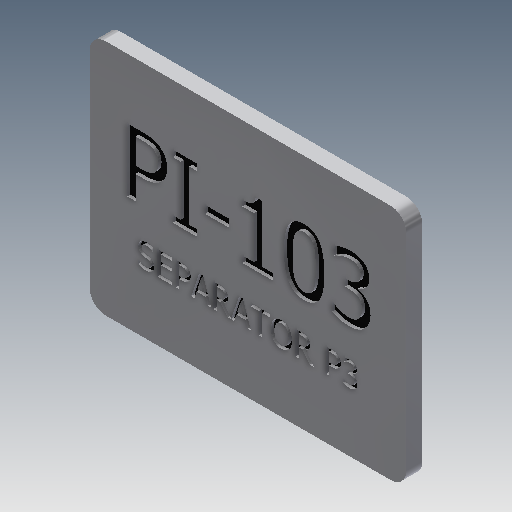
# Autodesk Inventor part: PI-103_Instrument Name Plate
Saved by Autodesk Inventor 2019.1 (Build 231200000, 200)
## iProperties
Created: 2009-08-11
Part Number: PI-103_Instrument Name Plate
Material: Polyaryletherketone Resin
Document SubType Name: Modeling
Designer: Demir Ali
Mass: 48.4644 g
Surface Area: 174.794 cm^2
Volume: 36.7154 cm^3
Density: 1.32 g/cm^3
Description: Name Plate
Stock Number: NA
Appearance: Smooth - White
Title: Purchased Part
Author: Demir Ali
Revision Number: A
Autodesk Inventor part; units mm, degrees
ref_plane "YZ Plane" through (0, 0, 0) normal (1, 0, 0) x (0, 1, 0)
ref_plane "XZ Plane" through (0, 0, 0) normal (0, 1, 0) x (-1, 0, 0)
ref_plane "XY Plane" through (0, 0, 0) normal (0, 0, 1) x (1, 0, 0)
sketch "Sketch1" plane through (0, 0, 0) normal (0, 0, 1) x (1, 0, 0)
  line L0 (-50, -37.5) -> (50, -37.5)
  line L1 (50, -37.5) -> (50, 37.5)
  line L2 (50, 37.5) -> (-50, 37.5)
  line L3 (-50, 37.5) -> (-50, -37.5)
  point P0 (0, 0)
  point P1 (50, 0)
  point P2 (0, 37.5)
  dimension "d0" = 100
  dimension "d1" = 75
  constraints: 8 end point, 2 midpoint, 2 parallel, 1 horizontal, 1 horizontal alignment, 1 perpendicular, 1 vertical alignment
  measures "d0" distance of L1.end L2.end
  measures "d1" distance of L0.end L1.end
extrude "Extrusion1" add sketch "Sketch1" along normal blind 5
sketch "Sketch2" plane through (0, 0, 5) normal (0, 0, 1) x (1, 0, 0)
  line L0 (-39.7109, 33.8079) -> (39.7109, 33.8079) construction
  line L1 (39.7109, 33.8079) -> (39.7109, -33.8079) construction
  line L2 (39.7109, -33.8079) -> (-39.7109, -33.8079) construction
  line L3 (-39.7109, -33.8079) -> (-39.7109, 33.8079) construction
  line L4 (-50, -37.5) -> (-50, 37.5) projected
  line L5 (50, -37.5) -> (-50, -37.5) projected
  line L6 (50, 37.5) -> (50, -37.5) projected
  line L7 (-50, 37.5) -> (50, 37.5) projected
  spline S0 degree 2 poles (-25.5511, 12.4253) (-25.5511, 11.1287) (-26.4749, 8.7948) (-27.3015, 7.9844) knots 0 0 0 1 2 2 2
  spline S1 degree 2 poles (-27.3015, 7.9844) (-28.3387, 6.9633) (-31.1426, 5.9099) (-33.282, 5.9099) knots 0 0 0 1 2 2 2
  line L8 (-33.282, 5.9099) -> (-35.5348, 5.9099)
  line L9 (-35.5348, 5.9099) -> (-35.5348, -1.5456)
  line L10 (-35.5348, -1.5456) -> (-38.1929, -1.5456)
  line L11 (-38.1929, -1.5456) -> (-38.1929, 18.4544)
  line L12 (-38.1929, 18.4544) -> (-33.1686, 18.4544)
  spline S2 degree 2 poles (-33.1686, 18.4544) (-31.3857, 18.4544) (-28.8898, 17.871) (-27.9336, 17.2065) knots 0 0 0 1 2 2 2
  spline S3 degree 2 poles (-27.9336, 17.2065) (-26.8152, 16.4447) (-25.5511, 14.0946) (-25.5511, 12.4253) knots 0 0 0 1 2 2 2
  spline S4 degree 2 poles (-28.3225, 12.3442) (-28.3225, 13.3815) (-29.0357, 14.905) (-29.765, 15.3912) knots 0 0 0 1 2 2 2
  spline S5 degree 2 poles (-29.765, 15.3912) (-30.3971, 15.8126) (-32.0827, 16.153) (-33.3306, 16.153) knots 0 0 0 1 2 2 2
  line L13 (-33.3306, 16.153) -> (-35.5348, 16.153)
  line L14 (-35.5348, 16.153) -> (-35.5348, 8.1789)
  line L15 (-35.5348, 8.1789) -> (-33.7196, 8.1789)
  spline S6 degree 2 poles (-33.7196, 8.1789) (-32.0989, 8.1789) (-30.1053, 8.6975) (-29.4571, 9.3783) knots 0 0 0 1 2 2 2
  spline S7 degree 2 poles (-29.4571, 9.3783) (-28.8574, 9.9779) (-28.3225, 11.388) (-28.3225, 12.3442) knots 0 0 0 1 2 2 2
  line L16 (-16.0535, -1.5456) -> (-23.8006, -1.5456)
  line L17 (-23.8006, -1.5456) -> (-23.8006, 0.4966)
  line L18 (-23.8006, 0.4966) -> (-21.2561, 0.4966)
  line L19 (-21.2561, 0.4966) -> (-21.2561, 16.4123)
  line L20 (-21.2561, 16.4123) -> (-23.8006, 16.4123)
  line L21 (-23.8006, 16.4123) -> (-23.8006, 18.4544)
  line L22 (-23.8006, 18.4544) -> (-16.0535, 18.4544)
  line L23 (-16.0535, 18.4544) -> (-16.0535, 16.4123)
  line L24 (-16.0535, 16.4123) -> (-18.5981, 16.4123)
  line L25 (-18.5981, 16.4123) -> (-18.5981, 0.4966)
  line L26 (-18.5981, 0.4966) -> (-16.0535, 0.4966)
  line L27 (-16.0535, 0.4966) -> (-16.0535, -1.5456)
  line L28 (-6.0049, 5.9909) -> (-13.5737, 5.9909)
  line L29 (-13.5737, 5.9909) -> (-13.5737, 8.422)
  line L30 (-13.5737, 8.422) -> (-6.0049, 8.422)
  line L31 (-6.0049, 8.422) -> (-6.0049, 5.9909)
  line L32 (7.9822, -1.5456) -> (-1.7747, -1.5456)
  line L33 (-1.7747, -1.5456) -> (-1.7747, 0.4966)
  line L34 (-1.7747, 0.4966) -> (1.8558, 0.4966)
  line L35 (1.8558, 0.4966) -> (1.8558, 13.9001)
  line L36 (1.8558, 13.9001) -> (-1.7747, 13.9001)
  line L37 (-1.7747, 13.9001) -> (-1.7747, 15.7316)
  spline S8 degree 2 poles (-1.7747, 15.7316) (0.2836, 15.7316) (2.2285, 16.8985) (2.3582, 18.5193) knots 0 0 0 1 2 2 2
  line L38 (2.3582, 18.5193) -> (4.4327, 18.5193)
  line L39 (4.4327, 18.5193) -> (4.4327, 0.4966)
  line L40 (4.4327, 0.4966) -> (7.9822, 0.4966)
  line L41 (7.9822, 0.4966) -> (7.9822, -1.5456)
  spline S9 degree 2 poles (24.1086, 8.4544) (24.1086, 3.0736) (20.9806, -1.967) (17.7229, -1.967) knots 0 0 0 1 2 2 2
  spline S10 degree 2 poles (17.7229, -1.967) (14.4165, -1.967) (11.3209, 3.1708) (11.3209, 8.4382) knots 0 0 0 1 2 2 2
  spline S11 degree 2 poles (11.3209, 8.4382) (11.3209, 13.8515) (14.4489, 18.8596) (17.7229, 18.8596) knots 0 0 0 1 2 2 2
  spline S12 degree 2 poles (17.7229, 18.8596) (21.013, 18.8596) (24.1086, 13.6732) (24.1086, 8.4544) knots 0 0 0 1 2 2 2
  spline S13 degree 2 poles (20.6726, 2.3604) (21.0616, 3.3491) (21.3857, 6.3961) (21.3857, 8.4544) knots 0 0 0 1 2 2 2
  spline S14 degree 2 poles (21.3857, 8.4544) (21.3857, 10.5128) (21.0616, 13.5436) (20.6564, 14.5646) knots 0 0 0 1 2 2 2
  spline S15 degree 2 poles (20.6564, 14.5646) (20.2512, 15.5857) (18.8412, 16.6392) (17.7229, 16.6392) knots 0 0 0 1 2 2 2
  spline S16 degree 2 poles (17.7229, 16.6392) (16.6045, 16.6392) (15.1621, 15.5857) (14.7407, 14.5322) knots 0 0 0 1 2 2 2
  spline S17 degree 2 poles (14.7407, 14.5322) (14.3355, 13.5112) (14.0438, 10.3993) (14.0438, 8.4382) knots 0 0 0 1 2 2 2
  spline S18 degree 2 poles (14.0438, 8.4382) (14.0438, 6.3313) (14.3031, 3.5112) (14.7245, 2.4091) knots 0 0 0 1 2 2 2
  spline S19 degree 2 poles (14.7245, 2.4091) (15.1135, 1.3718) (16.5559, 0.2535) (17.7229, 0.2535) knots 0 0 0 1 2 2 2
  spline S20 degree 2 poles (17.7229, 0.2535) (18.825, 0.2535) (20.2674, 1.3069) (20.6726, 2.3604) knots 0 0 0 1 2 2 2
  spline S21 degree 2 poles (32.0664, 16.5582) (31.3371, 16.5582) (29.8947, 16.2016) (29.1977, 15.9261) knots 0 0 0 1 2 2 2
  spline S22 degree 2 poles (29.1977, 15.9261) (28.5494, 15.6505) (27.5932, 15.0671) (27.2204, 14.8078) knots 0 0 0 1 2 2 2
  line L42 (27.2204, 14.8078) -> (27.0583, 14.8078)
  line L43 (27.0583, 14.8078) -> (27.0583, 17.6441)
  spline S23 degree 2 poles (27.0583, 17.6441) (27.9335, 18.1141) (30.9319, 18.8758) (32.2771, 18.8758) knots 0 0 0 1 2 2 2
  spline S24 degree 2 poles (32.2771, 18.8758) (33.6386, 18.8758) (35.6645, 18.3248) (36.4911, 17.7413) knots 0 0 0 1 2 2 2
  spline S25 degree 2 poles (36.4911, 17.7413) (37.3663, 17.1092) (38.2739, 15.2778) (38.2739, 14.046) knots 0 0 0 1 2 2 2
  spline S26 degree 2 poles (38.2739, 14.046) (38.2739, 12.3928) (36.1021, 9.8969) (34.5786, 9.5727) knots 0 0 0 1 2 2 2
  line L44 (34.5786, 9.5727) -> (34.5786, 9.3783)
  spline S27 degree 2 poles (34.5786, 9.3783) (35.2107, 9.2486) (36.6532, 8.6651) (37.269, 8.0817) knots 0 0 0 1 2 2 2
  spline S28 degree 2 poles (37.269, 8.0817) (37.8849, 7.5144) (38.6629, 5.6992) (38.6629, 4.3864) knots 0 0 0 1 2 2 2
  spline S29 degree 2 poles (38.6629, 4.3864) (38.6629, 3.0411) (37.7391, 0.7559) (36.8963, -0.1193) knots 0 0 0 1 2 2 2
  spline S30 degree 2 poles (36.8963, -0.1193) (36.0211, -1.0269) (33.5413, -1.967) (31.9692, -1.967) knots 0 0 0 1 2 2 2
  spline S31 degree 2 poles (31.9692, -1.967) (30.4619, -1.967) (27.5122, -1.2376) (26.5073, -0.7352) knots 0 0 0 1 2 2 2
  line L45 (26.5073, -0.7352) -> (26.5073, 2.1011)
  line L46 (26.5073, 2.1011) -> (26.7018, 2.1011)
  spline S32 degree 2 poles (26.7018, 2.1011) (27.5446, 1.4852) (30.3971, 0.3507) (31.8071, 0.3507) knots 0 0 0 1 2 2 2
  spline S33 degree 2 poles (31.8071, 0.3507) (32.6337, 0.3507) (34.2869, 0.8693) (34.8379, 1.469) knots 0 0 0 1 2 2 2
  spline S34 degree 2 poles (34.8379, 1.469) (35.3728, 2.0687) (35.94, 3.495) (35.94, 4.5809) knots 0 0 0 1 2 2 2
  spline S35 degree 2 poles (35.94, 4.5809) (35.94, 5.6668) (35.3079, 7.0768) (34.7407, 7.482) knots 0 0 0 1 2 2 2
  spline S36 degree 2 poles (34.7407, 7.482) (34.1734, 7.8872) (32.6337, 8.1951) (31.7261, 8.1951) knots 0 0 0 1 2 2 2
  line L47 (31.7261, 8.1951) -> (30.5916, 8.1951)
  line L48 (30.5916, 8.1951) -> (30.5916, 10.4155)
  line L49 (30.5916, 10.4155) -> (31.483, 10.4155)
  spline S37 degree 2 poles (31.483, 10.4155) (33.282, 10.4155) (35.5511, 12.1335) (35.5511, 13.7705) knots 0 0 0 1 2 2 2
  spline S38 degree 2 poles (35.5511, 13.7705) (35.5511, 14.5322) (34.9676, 15.6181) (34.4976, 15.9423) knots 0 0 0 1 2 2 2
  spline S39 degree 2 poles (34.4976, 15.9423) (33.9951, 16.2826) (32.7634, 16.5582) (32.0664, 16.5582) knots 0 0 0 1 2 2 2
  spline S40 degree 2 poles (-32.2761, -18.8515) (-33.0906, -18.8515) (-34.2332, -18.5112) (-34.7376, -18.268) knots 0 0 0 1 2 2 2
  line L50 (-34.7376, -18.268) -> (-34.7376, -17.016)
  line L51 (-34.7376, -17.016) -> (-34.6647, -17.016)
  spline S41 degree 2 poles (-34.6647, -17.016) (-34.1724, -17.4779) (-32.9265, -17.9885) (-32.3491, -17.9885) knots 0 0 0 1 2 2 2
  spline S42 degree 2 poles (-32.3491, -17.9885) (-31.5225, -17.9885) (-30.6777, -17.3017) (-30.6777, -16.7364) knots 0 0 0 1 2 2 2
  spline S43 degree 2 poles (-30.6777, -16.7364) (-30.6777, -16.2867) (-31.1214, -15.7275) (-31.6015, -15.5877) knots 0 0 0 1 2 2 2
  spline S44 degree 2 poles (-31.6015, -15.5877) (-31.9479, -15.4905) (-32.5253, -15.3568) (-32.9568, -15.2474) knots 0 0 0 1 2 2 2
  spline S45 degree 2 poles (-32.9568, -15.2474) (-33.3458, -15.1441) (-33.9597, -14.8341) (-34.1967, -14.5849) knots 0 0 0 1 2 2 2
  spline S46 degree 2 poles (-34.1967, -14.5849) (-34.4277, -14.3357) (-34.6829, -13.6672) (-34.6829, -13.2296) knots 0 0 0 1 2 2 2
  spline S47 degree 2 poles (-34.6829, -13.2296) (-34.6829, -12.3179) (-33.2607, -11.0841) (-32.1607, -11.0841) knots 0 0 0 1 2 2 2
  spline S48 degree 2 poles (-32.1607, -11.0841) (-31.5286, -11.0841) (-30.4103, -11.3333) (-29.9301, -11.5703) knots 0 0 0 1 2 2 2
  line L52 (-29.9301, -11.5703) -> (-29.9301, -12.7616)
  line L53 (-29.9301, -12.7616) -> (-30.003, -12.7616)
  spline S49 degree 2 poles (-30.003, -12.7616) (-30.3616, -12.4334) (-31.4799, -11.9471) (-32.0938, -11.9471) knots 0 0 0 1 2 2 2
  spline S50 degree 2 poles (-32.0938, -11.9471) (-32.7867, -11.9471) (-33.6436, -12.5975) (-33.6436, -13.1262) knots 0 0 0 1 2 2 2
  spline S51 degree 2 poles (-33.6436, -13.1262) (-33.6436, -13.6003) (-33.1392, -14.1655) (-32.6651, -14.2932) knots 0 0 0 1 2 2 2
  spline S52 degree 2 poles (-32.6651, -14.2932) (-32.3491, -14.3783) (-31.4313, -14.5971) (-31.1274, -14.6882) knots 0 0 0 1 2 2 2
  spline S53 degree 2 poles (-31.1274, -14.6882) (-30.3556, -14.9253) (-29.6384, -15.8795) (-29.6384, -16.5784) knots 0 0 0 1 2 2 2
  spline S54 degree 2 poles (-29.6384, -16.5784) (-29.6384, -17.0221) (-29.997, -17.873) (-30.3191, -18.1708) knots 0 0 0 1 2 2 2
  spline S55 degree 2 poles (-30.3191, -18.1708) (-30.6777, -18.499) (-31.5893, -18.8515) (-32.2761, -18.8515) knots 0 0 0 1 2 2 2
  line L54 (-28.6234, -18.7178) -> (-28.6234, -11.2178)
  line L55 (-28.6234, -11.2178) -> (-23.9313, -11.2178)
  line L56 (-23.9313, -11.2178) -> (-23.9313, -12.1052)
  line L57 (-23.9313, -12.1052) -> (-27.6266, -12.1052)
  line L58 (-27.6266, -12.1052) -> (-27.6266, -14.1595)
  line L59 (-27.6266, -14.1595) -> (-24.1805, -14.1595)
  line L60 (-24.1805, -14.1595) -> (-24.1805, -15.0468)
  line L61 (-24.1805, -15.0468) -> (-27.6266, -15.0468)
  line L62 (-27.6266, -15.0468) -> (-27.6266, -17.8304)
  line L63 (-27.6266, -17.8304) -> (-23.9313, -17.8304)
  line L64 (-23.9313, -17.8304) -> (-23.9313, -18.7178)
  line L65 (-23.9313, -18.7178) -> (-28.6234, -18.7178)
  spline S56 degree 2 poles (-18.0966, -13.4787) (-18.0966, -13.965) (-18.4431, -14.8402) (-18.753, -15.1441) knots 0 0 0 1 2 2 2
  spline S57 degree 2 poles (-18.753, -15.1441) (-19.142, -15.527) (-20.1935, -15.922) (-20.9957, -15.922) knots 0 0 0 1 2 2 2
  line L66 (-20.9957, -15.922) -> (-21.8406, -15.922)
  line L67 (-21.8406, -15.922) -> (-21.8406, -18.7178)
  line L68 (-21.8406, -18.7178) -> (-22.8373, -18.7178)
  line L69 (-22.8373, -18.7178) -> (-22.8373, -11.2178)
  line L70 (-22.8373, -11.2178) -> (-20.9532, -11.2178)
  spline S58 degree 2 poles (-20.9532, -11.2178) (-20.2846, -11.2178) (-19.3487, -11.4366) (-18.9901, -11.6858) knots 0 0 0 1 2 2 2
  spline S59 degree 2 poles (-18.9901, -11.6858) (-18.5707, -11.9714) (-18.0966, -12.8527) (-18.0966, -13.4787) knots 0 0 0 1 2 2 2
  spline S60 degree 2 poles (-19.1359, -13.5091) (-19.1359, -13.1202) (-19.4034, -12.5488) (-19.6769, -12.3665) knots 0 0 0 1 2 2 2
  spline S61 degree 2 poles (-19.6769, -12.3665) (-19.9139, -12.2085) (-20.546, -12.0808) (-21.014, -12.0808) knots 0 0 0 1 2 2 2
  line L71 (-21.014, -12.0808) -> (-21.8406, -12.0808)
  line L72 (-21.8406, -12.0808) -> (-21.8406, -15.0711)
  line L73 (-21.8406, -15.0711) -> (-21.1598, -15.0711)
  spline S62 degree 2 poles (-21.1598, -15.0711) (-20.5521, -15.0711) (-19.8045, -14.8766) (-19.5614, -14.6214) knots 0 0 0 1 2 2 2
  spline S63 degree 2 poles (-19.5614, -14.6214) (-19.3365, -14.3965) (-19.1359, -13.8677) (-19.1359, -13.5091) knots 0 0 0 1 2 2 2
  line L74 (-17.9568, -18.7178) -> (-15.4285, -11.2178)
  line L75 (-15.4285, -11.2178) -> (-14.2008, -11.2178)
  line L76 (-14.2008, -11.2178) -> (-11.6724, -18.7178)
  line L77 (-11.6724, -18.7178) -> (-12.7239, -18.7178)
  line L78 (-12.7239, -18.7178) -> (-13.4046, -16.621)
  line L79 (-13.4046, -16.621) -> (-16.2672, -16.621)
  line L80 (-16.2672, -16.621) -> (-16.9479, -18.7178)
  line L81 (-16.9479, -18.7178) -> (-17.9568, -18.7178)
  line L82 (-13.6781, -15.7701) -> (-14.8389, -12.2389)
  line L83 (-14.8389, -12.2389) -> (-15.9937, -15.7701)
  line L84 (-15.9937, -15.7701) -> (-13.6781, -15.7701)
  line L85 (-5.157, -18.7178) -> (-6.4516, -18.7178)
  line L86 (-6.4516, -18.7178) -> (-8.8219, -15.7336)
  line L87 (-8.8219, -15.7336) -> (-9.9645, -15.7336)
  line L88 (-9.9645, -15.7336) -> (-9.9645, -18.7178)
  line L89 (-9.9645, -18.7178) -> (-10.9613, -18.7178)
  line L90 (-10.9613, -18.7178) -> (-10.9613, -11.2178)
  line L91 (-10.9613, -11.2178) -> (-9.0286, -11.2178)
  spline S64 degree 2 poles (-9.0286, -11.2178) (-8.3843, -11.2178) (-7.5152, -11.3576) (-7.1201, -11.6129) knots 0 0 0 1 2 2 2
  spline S65 degree 2 poles (-7.1201, -11.6129) (-6.7251, -11.8681) (-6.2692, -12.6643) (-6.2692, -13.2539) knots 0 0 0 1 2 2 2
  spline S66 degree 2 poles (-6.2692, -13.2539) (-6.2692, -14.0744) (-7.108, -15.1866) (-7.8252, -15.454) knots 0 0 0 1 2 2 2
  line L92 (-7.8252, -15.454) -> (-5.157, -18.7178)
  spline S67 degree 2 poles (-7.3086, -13.3329) (-7.3086, -13.0047) (-7.5395, -12.5002) (-7.7826, -12.3361) knots 0 0 0 1 2 2 2
  spline S68 degree 2 poles (-7.7826, -12.3361) (-7.9953, -12.1963) (-8.5606, -12.0808) (-8.9739, -12.0808) knots 0 0 0 1 2 2 2
  line L93 (-8.9739, -12.0808) -> (-9.9645, -12.0808)
  line L94 (-9.9645, -12.0808) -> (-9.9645, -14.9009)
  line L95 (-9.9645, -14.9009) -> (-9.0893, -14.9009)
  spline S69 degree 2 poles (-9.0893, -14.9009) (-8.6578, -14.9009) (-7.971, -14.749) (-7.734, -14.512) knots 0 0 0 1 2 2 2
  spline S70 degree 2 poles (-7.734, -14.512) (-7.5152, -14.3053) (-7.3086, -13.7219) (-7.3086, -13.3329) knots 0 0 0 1 2 2 2
  line L96 (-5.3697, -18.7178) -> (-2.8414, -11.2178)
  line L97 (-2.8414, -11.2178) -> (-1.6137, -11.2178)
  line L98 (-1.6137, -11.2178) -> (0.9147, -18.7178)
  line L99 (0.9147, -18.7178) -> (-0.1368, -18.7178)
  line L100 (-0.1368, -18.7178) -> (-0.8175, -16.621)
  line L101 (-0.8175, -16.621) -> (-3.6801, -16.621)
  line L102 (-3.6801, -16.621) -> (-4.3608, -18.7178)
  line L103 (-4.3608, -18.7178) -> (-5.3697, -18.7178)
  line L104 (-1.091, -15.7701) -> (-2.2518, -12.2389)
  line L105 (-2.2518, -12.2389) -> (-3.4066, -15.7701)
  line L106 (-3.4066, -15.7701) -> (-1.091, -15.7701)
  line L107 (3.3762, -18.7178) -> (3.3762, -12.1052)
  line L108 (3.3762, -12.1052) -> (0.86, -12.1052)
  line L109 (0.86, -12.1052) -> (0.86, -11.2178)
  line L110 (0.86, -11.2178) -> (6.8892, -11.2178)
  line L111 (6.8892, -11.2178) -> (6.8892, -12.1052)
  line L112 (6.8892, -12.1052) -> (4.373, -12.1052)
  line L113 (4.373, -12.1052) -> (4.373, -18.7178)
  line L114 (4.373, -18.7178) -> (3.3762, -18.7178)
  spline S71 degree 2 poles (12.9548, -12.0748) (13.3803, -12.5732) (13.8543, -14.0318) (13.8543, -14.9678) knots 0 0 0 1 2 2 2
  spline S72 degree 2 poles (13.8543, -14.9678) (13.8543, -15.8795) (13.3924, -17.3564) (12.9548, -17.8548) knots 0 0 0 1 2 2 2
  spline S73 degree 2 poles (12.9548, -17.8548) (12.4929, -18.3774) (11.2713, -18.8758) (10.5359, -18.8758) knots 0 0 0 1 2 2 2
  spline S74 degree 2 poles (10.5359, -18.8758) (9.7761, -18.8758) (8.5606, -18.3592) (8.1169, -17.8548) knots 0 0 0 1 2 2 2
  spline S75 degree 2 poles (8.1169, -17.8548) (7.6854, -17.3564) (7.2235, -15.8916) (7.2235, -14.9678) knots 0 0 0 1 2 2 2
  spline S76 degree 2 poles (7.2235, -14.9678) (7.2235, -14.0257) (7.6914, -12.5914) (8.123, -12.0748) knots 0 0 0 1 2 2 2
  spline S77 degree 2 poles (8.123, -12.0748) (8.5606, -11.5764) (9.7822, -11.0598) (10.5359, -11.0598) knots 0 0 0 1 2 2 2
  spline S78 degree 2 poles (10.5359, -11.0598) (11.3017, -11.0598) (12.5294, -11.5946) (12.9548, -12.0748) knots 0 0 0 1 2 2 2
  spline S79 degree 2 poles (12.815, -14.9678) (12.815, -14.2263) (12.4929, -13.0776) (12.2012, -12.7008) knots 0 0 0 1 2 2 2
  spline S80 degree 2 poles (12.2012, -12.7008) (11.9034, -12.3118) (11.0646, -11.9228) (10.5419, -11.9228) knots 0 0 0 1 2 2 2
  spline S81 degree 2 poles (10.5419, -11.9228) (10.001, -11.9228) (9.1866, -12.2997) (8.8766, -12.7008) knots 0 0 0 1 2 2 2
  spline S82 degree 2 poles (8.8766, -12.7008) (8.5788, -13.0837) (8.2628, -14.2385) (8.2628, -14.9678) knots 0 0 0 1 2 2 2
  spline S83 degree 2 poles (8.2628, -14.9678) (8.2628, -16.4447) (9.5026, -18.0128) (10.5419, -18.0128) knots 0 0 0 1 2 2 2
  spline S84 degree 2 poles (10.5419, -18.0128) (11.5812, -18.0128) (12.815, -16.4447) (12.815, -14.9678) knots 0 0 0 1 2 2 2
  line L115 (20.7526, -18.7178) -> (19.4581, -18.7178)
  line L116 (19.4581, -18.7178) -> (17.0877, -15.7336)
  line L117 (17.0877, -15.7336) -> (15.9451, -15.7336)
  line L118 (15.9451, -15.7336) -> (15.9451, -18.7178)
  line L119 (15.9451, -18.7178) -> (14.9483, -18.7178)
  line L120 (14.9483, -18.7178) -> (14.9483, -11.2178)
  line L121 (14.9483, -11.2178) -> (16.8811, -11.2178)
  spline S85 degree 2 poles (16.8811, -11.2178) (17.5253, -11.2178) (18.3944, -11.3576) (18.7895, -11.6129) knots 0 0 0 1 2 2 2
  spline S86 degree 2 poles (18.7895, -11.6129) (19.1846, -11.8681) (19.6404, -12.6643) (19.6404, -13.2539) knots 0 0 0 1 2 2 2
  spline S87 degree 2 poles (19.6404, -13.2539) (19.6404, -14.0744) (18.8017, -15.1866) (18.0845, -15.454) knots 0 0 0 1 2 2 2
  line L122 (18.0845, -15.454) -> (20.7526, -18.7178)
  spline S88 degree 2 poles (18.6011, -13.3329) (18.6011, -13.0047) (18.3701, -12.5002) (18.127, -12.3361) knots 0 0 0 1 2 2 2
  spline S89 degree 2 poles (18.127, -12.3361) (17.9143, -12.1963) (17.3491, -12.0808) (16.9358, -12.0808) knots 0 0 0 1 2 2 2
  line L123 (16.9358, -12.0808) -> (15.9451, -12.0808)
  line L124 (15.9451, -12.0808) -> (15.9451, -14.9009)
  line L125 (15.9451, -14.9009) -> (16.8203, -14.9009)
  spline S90 degree 2 poles (16.8203, -14.9009) (17.2518, -14.9009) (17.9386, -14.749) (18.1756, -14.512) knots 0 0 0 1 2 2 2
  spline S91 degree 2 poles (18.1756, -14.512) (18.3944, -14.3053) (18.6011, -13.7219) (18.6011, -13.3329) knots 0 0 0 1 2 2 2
  spline S92 degree 2 poles (29.3102, -13.4787) (29.3102, -13.965) (28.9637, -14.8402) (28.6538, -15.1441) knots 0 0 0 1 2 2 2
  spline S93 degree 2 poles (28.6538, -15.1441) (28.2648, -15.527) (27.2133, -15.922) (26.4111, -15.922) knots 0 0 0 1 2 2 2
  line L126 (26.4111, -15.922) -> (25.5662, -15.922)
  line L127 (25.5662, -15.922) -> (25.5662, -18.7178)
  line L128 (25.5662, -18.7178) -> (24.5695, -18.7178)
  line L129 (24.5695, -18.7178) -> (24.5695, -11.2178)
  line L130 (24.5695, -11.2178) -> (26.4536, -11.2178)
  spline S94 degree 2 poles (26.4536, -11.2178) (27.1222, -11.2178) (28.0581, -11.4366) (28.4167, -11.6858) knots 0 0 0 1 2 2 2
  spline S95 degree 2 poles (28.4167, -11.6858) (28.8361, -11.9714) (29.3102, -12.8527) (29.3102, -13.4787) knots 0 0 0 1 2 2 2
  spline S96 degree 2 poles (28.2709, -13.5091) (28.2709, -13.1202) (28.0034, -12.5488) (27.7299, -12.3665) knots 0 0 0 1 2 2 2
  spline S97 degree 2 poles (27.7299, -12.3665) (27.4929, -12.2085) (26.8608, -12.0808) (26.3928, -12.0808) knots 0 0 0 1 2 2 2
  line L131 (26.3928, -12.0808) -> (25.5662, -12.0808)
  line L132 (25.5662, -12.0808) -> (25.5662, -15.0711)
  line L133 (25.5662, -15.0711) -> (26.247, -15.0711)
  spline S98 degree 2 poles (26.247, -15.0711) (26.8547, -15.0711) (27.6023, -14.8766) (27.8454, -14.6214) knots 0 0 0 1 2 2 2
  spline S99 degree 2 poles (27.8454, -14.6214) (28.0703, -14.3965) (28.2709, -13.8677) (28.2709, -13.5091) knots 0 0 0 1 2 2 2
  spline S100 degree 2 poles (32.0695, -11.9289) (31.796, -11.9289) (31.2551, -12.0626) (30.9937, -12.1659) knots 0 0 0 1 2 2 2
  spline S101 degree 2 poles (30.9937, -12.1659) (30.7506, -12.2693) (30.392, -12.4881) (30.2522, -12.5853) knots 0 0 0 1 2 2 2
  line L134 (30.2522, -12.5853) -> (30.1914, -12.5853)
  line L135 (30.1914, -12.5853) -> (30.1914, -11.5217)
  spline S102 degree 2 poles (30.1914, -11.5217) (30.5197, -11.3454) (31.644, -11.0598) (32.1485, -11.0598) knots 0 0 0 1 2 2 2
  spline S103 degree 2 poles (32.1485, -11.0598) (32.659, -11.0598) (33.4188, -11.2664) (33.7287, -11.4852) knots 0 0 0 1 2 2 2
  spline S104 degree 2 poles (33.7287, -11.4852) (34.0569, -11.7223) (34.3973, -12.4091) (34.3973, -12.871) knots 0 0 0 1 2 2 2
  spline S105 degree 2 poles (34.3973, -12.871) (34.3973, -13.4909) (33.5829, -14.4269) (33.0115, -14.5484) knots 0 0 0 1 2 2 2
  line L136 (33.0115, -14.5484) -> (33.0115, -14.6214)
  spline S106 degree 2 poles (33.0115, -14.6214) (33.2486, -14.67) (33.7895, -14.8888) (34.0205, -15.1076) knots 0 0 0 1 2 2 2
  spline S107 degree 2 poles (34.0205, -15.1076) (34.2514, -15.3203) (34.5432, -16.001) (34.5432, -16.4933) knots 0 0 0 1 2 2 2
  spline S108 degree 2 poles (34.5432, -16.4933) (34.5432, -16.9978) (34.1967, -17.8548) (33.8807, -18.183) knots 0 0 0 1 2 2 2
  spline S109 degree 2 poles (33.8807, -18.183) (33.5525, -18.5233) (32.6226, -18.8758) (32.033, -18.8758) knots 0 0 0 1 2 2 2
  spline S110 degree 2 poles (32.033, -18.8758) (31.4678, -18.8758) (30.3616, -18.6023) (29.9848, -18.4139) knots 0 0 0 1 2 2 2
  line L137 (29.9848, -18.4139) -> (29.9848, -17.3503)
  line L138 (29.9848, -17.3503) -> (30.0577, -17.3503)
  spline S111 degree 2 poles (30.0577, -17.3503) (30.3738, -17.5813) (31.4435, -18.0067) (31.9722, -18.0067) knots 0 0 0 1 2 2 2
  spline S112 degree 2 poles (31.9722, -18.0067) (32.2822, -18.0067) (32.9021, -17.8122) (33.1088, -17.5873) knots 0 0 0 1 2 2 2
  spline S113 degree 2 poles (33.1088, -17.5873) (33.3094, -17.3625) (33.5221, -16.8276) (33.5221, -16.4204) knots 0 0 0 1 2 2 2
  spline S114 degree 2 poles (33.5221, -16.4204) (33.5221, -16.0132) (33.285, -15.4844) (33.0723, -15.3325) knots 0 0 0 1 2 2 2
  spline S115 degree 2 poles (33.0723, -15.3325) (32.8596, -15.1805) (32.2822, -15.065) (31.9419, -15.065) knots 0 0 0 1 2 2 2
  line L139 (31.9419, -15.065) -> (31.5164, -15.065)
  line L140 (31.5164, -15.065) -> (31.5164, -14.2324)
  line L141 (31.5164, -14.2324) -> (31.8507, -14.2324)
  spline S116 degree 2 poles (31.8507, -14.2324) (32.5253, -14.2324) (33.3762, -13.5881) (33.3762, -12.9743) knots 0 0 0 1 2 2 2
  spline S117 degree 2 poles (33.3762, -12.9743) (33.3762, -12.6886) (33.1574, -12.2814) (32.9812, -12.1599) knots 0 0 0 1 2 2 2
  spline S118 degree 2 poles (32.9812, -12.1599) (32.7927, -12.0322) (32.3308, -11.9289) (32.0695, -11.9289) knots 0 0 0 1 2 2 2
  point P0 (0, 0)
  point P1 (0, 33.8079)
  point P2 (-39.7109, 0)
  constraints: 2 midpoint, 1 horizontal alignment, 1 vertical alignment, 2 other
emboss "Emboss1" sketch "Sketch2" operation cut depth 1 direction (0, 0, -1) contours S0 S1 L8 L9 L10 L11 L12 S2 S3 | L16 L17 L18 L19 L20 L21 L22 L23 L24 L25 L26 L27 | L28 L29 L30 L31 | L32 L33 L34 L35 L36 L37 S8 L38 L39 L40 L41 | S9 S10 S11 S12 | S21 S22 L42 L43 S23 S24 S25 S26 L44 S27 S28 S29 S30 S31 L45 L46 S32 S33 S34 S35 S36 L47 L48 L49 S37 S38 S39 | S40 L50 L51 S41 S42 S43 S44 S45 S46 S47 S48 L52 L53 S49 S50 S51 S52 S53 S54 S55 | L54 L55 L56 L57 L58 L59 L60 L61 L62 L63 L64 L65 | S56 S57 L66 L67 L68 L69 L70 S58 S59 | L74 L75 L76 L77 L78 L79 L80 L81 | L85 L96 L92 | L92 L96 L97 L98 L99 L100 L101 L102 L103 | L85 L86 L87 L88 L89 L90 L91 S64 S65 S66 L92 L96 | L107 L108 L109 L110 L111 L112 L113 L114 | S71 S72 S73 S74 S75 S76 S77 S78 | L115 L116 L117 L118 L119 L120 L121 S85 S86 S87 L122 | S92 S93 L126 L127 L128 L129 L130 S94 S95 | S100 S101 L134 L135 S102 S103 S104 S105 L136 S106 S107 S108 S109 S110 L137 L138 S111 S112 S113 S114 S115 L139 L140 L141 S116 S117 S118
fillet "Fillet1" radius 5 4 edges at (-50, 37.5, 2.5) (50, 37.5, 2.5) (-50, -37.5, 2.5) (50, -37.5, 2.5)
body "Solid1"
